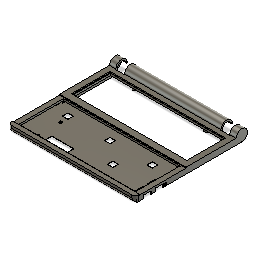
C_case (Autodesk Fusion 360 design; units mm, degrees)
Autodesk Fusion 360 part; units mm, degrees
sketch "Sketch1" plane through (0, 0, 0) normal (0, 1, 0) x (1, 0, 0)
  line L0 (0, 0) -> (230.6, 0)
  line L1 (230.6, 0) -> (230.6, 183)
  line L2 (230.6, 183) -> (0, 183)
  line L3 (0, 183) -> (0, 0)
  dimension "d1" = 230.6
  dimension "d2" = 183
  constraint horizontal L0
  constraint vertical L1
  constraint horizontal L2
  constraint vertical L3
  constraint coincident L0.start L3.end
  measures "d1" distance of L0.start L0.end
  measures "d2" distance of L0.start L2.end
extrude "Extrude1" add sketch "Sketch1" along normal blind 11
sketch "Sketch2" plane through (0, 11, 0) normal (0, 1, 0) x (-1, 0, 0)
  line L0 (0, 0) -> (-230.6, 0)
  line L1 (-230.6, -183) -> (0, -183)
  line L2 (-9, -10) -> (-221.6, -10)
  line L3 (-221.6, -10) -> (-221.6, -91.1)
  line L4 (-221.6, -91.1) -> (-9, -91.1)
  line L5 (-9, -91.1) -> (-9, -10)
  line L6 (-115.3, -77.3448) -> (-115.3, -22.2714) construction
  line L7 (0, -183) -> (0, 0)
  line L8 (-230.6, 0) -> (-230.6, -183)
  dimension "d5" = 212.6
  dimension "d6" = 81.1
  dimension "d7" = 10
  constraint horizontal L2
  constraint vertical L3
  constraint horizontal L4
  constraint vertical L5
  constraint perpendicular L1 L6
  constraint symmetric L3 L5 L6
  measures "d5" distance of L3.end L4.end
  measures "d6" distance of L2.start L4.end
  measures "d7" distance of L0 L2
extrude "Extrude2" cut sketch "Sketch2" against normal blind 5 contours L2 L3 L4 L5
sketch "Sketch3" plane through (0, 11, 0) normal (0, 1, 0) x (-1, 0, 0)
  line L0 (-221.6, -10) -> (-9, -10)
  line L1 (-9, -10) -> (-9, -91.1)
  line L2 (-9, -91.1) -> (-221.6, -91.1)
  line L3 (-221.6, -91.1) -> (-221.6, -10)
  line L4 (0, 0) -> (-230.6, 0)
  line L5 (-230.6, -183) -> (0, -183)
  line L6 (-10.05, -175) -> (-220.55, -175)
  line L7 (-220.55, -175) -> (-220.55, -104.5)
  line L8 (-220.55, -104.5) -> (-10.05, -104.5)
  line L9 (-10.05, -104.5) -> (-10.05, -175)
  line L10 (-115.3, -158.8) -> (-115.3, -113.8) construction
  line L11 (0, -183) -> (0, 0)
  line L12 (-230.6, 0) -> (-230.6, -183)
  dimension "d10" = 210.5
  dimension "d11" = 70.5
  dimension "d12" = 8
  constraint horizontal L6
  constraint vertical L7
  constraint horizontal L8
  constraint vertical L9
  constraint vertical L10
  constraint symmetric L7 L9 L10
  measures "d10" distance of L6.start L6.end
  measures "d11" distance of L6.start L8.end
  measures "d12" distance of L5 L6
extrude "Extrude3" cut sketch "Sketch3" against normal blind 1.95 contours L6 L7 L8 L9
sketch "Sketch4" plane through (0, 9.05, 0) normal (0, 1, 0) x (-1, 0, 0)
  line L0 (-10.05, -104.5) -> (-220.55, -104.5)
  line L1 (-220.55, -104.5) -> (-220.55, -175)
  line L2 (-220.55, -175) -> (-10.05, -175)
  line L3 (-10.05, -175) -> (-10.05, -104.5)
  line L4 (-11.55, -174.5) -> (-219.05, -174.5)
  line L5 (-219.05, -174.5) -> (-219.05, -105)
  line L6 (-219.05, -105) -> (-11.55, -105)
  line L7 (-11.55, -105) -> (-11.55, -174.5)
  dimension "d15" = 0.5
  dimension "d16" = 0.5
  dimension "d17" = 1.5
  dimension "d18" = 1.5
  constraint horizontal L4
  constraint vertical L5
  constraint horizontal L6
  constraint vertical L7
  measures "d15" distance of L2 L4
  measures "d16" distance of L0 L6
  measures "d17" distance of L3 L7
  measures "d18" distance of L1 L5
extrude "Extrude4" cut sketch "Sketch4" against normal blind 4.75 contours L4 L5 L6 L7
sketch "Sketch6" plane through (0, 0, 0) normal (-1, 0, 0) x (0, 0, 1)
  line L0 (-183, 0) -> (0, 0)
  line L1 (0, 0) -> (0, 11)
  line L2 (-183, 11) -> (-183, 0)
  line L3 (-8, 11) -> (-93, 11)
  line L4 (-93, 11) -> (-93, 9.5)
  line L5 (-93, 9.5) -> (-8, 9.5)
  line L6 (-8, 9.5) -> (-8, 11)
  line L7 (0, 11) -> (-183, 11)
  dimension "d26" = 1.5
  dimension "d27" = 85
  dimension "d28" = 8
  constraint horizontal L3
  constraint vertical L4
  constraint horizontal L5
  constraint vertical L6
  measures "d26" distance of L3.start L5.end
  measures "d27" distance of L3.start L3.end
  measures "d28" distance of L1 L6
extrude "Extrude6" cut sketch "Sketch6" against normal through all contours L3 L4 L5 L6 L7
sketch "Sketch8" plane through (0, 0, 0) normal (-1, 0, 0) x (0, 0, 1)
  line L0 (-183, 11) -> (-183, 0)
  line L1 (-183, 0) -> (0, 0)
  line L2 (0, 0) -> (0, 11)
  circle A0 centre (-194.5, 10.5) radius 10.5
  circle A1 centre (-194.5, 10.5) radius 9
  line L3 (-183, 0) -> (-194.5, 0)
  line L4 (-183, 0) -> (-184, 0)
  line L5 (-184, 0) -> (-184, 10.5)
  line L6 (-184, 10.5) -> (-183, 10.5)
  line L7 (-183, 10.5) -> (-183, 0)
  line L8 (-183, 11) -> (-184.0119, 11)
  line L9 (-93, 9.5) -> (-93, 11)
  line L10 (-93, 11) -> (-183, 11)
  line L11 (0, 11) -> (-8, 11)
  line L12 (-8, 11) -> (-8, 9.5)
  line L13 (-8, 9.5) -> (-93, 9.5)
  circle A2 centre (-194.5, 10.5) radius 7.5
  line L14 (-194.5, 10.5) -> (-203.5, 10.5)
  line L15 (-194.5, 10.5) -> (-202.7916, 14)
  dimension "d36" = 21
  dimension "d37" = 18
  dimension "d58" = 1
  dimension "d160" = 15
  dimension "d161" = 3.5
  constraint concentric A0 A1
  constraint coincident L0.end L1.start
  constraint coincident A0 L3.end
  constraint tangent A0 L3
  constraint parallel L1 L3
  constraint horizontal L4
  constraint vertical L5
  constraint horizontal L6
  constraint vertical L7
  constraint coincident A0 L5.end
  constraint tangent A0 L5
  constraint coincident L0.start L8.start
  constraint coincident A0 L8.end
  constraint perpendicular L0 L8
  constraint concentric A1 A2
  constraint coincident A0.centre A1.centre
  constraint coincident A1 L14.end
  constraint horizontal L14
  constraint coincident A1 L15.end
  measures "d36" diameter of A0
  measures "d37" diameter of A1
  measures "d58" distance of L5.end L6.end
  measures "d160" diameter of A2
  measures "d161" vertical distance of L14.end L15.end
extrude "Extrude7" add sketch "Sketch8" against normal blind 230.6 contours L0 A0 L6 L8 | L0 L3 L4 L5 L6 L7 | A0 | A1 A2 L14 L15 picked at (-186.0614, 9.6803)
extrude "Extrude8" add sketch "Sketch8" against normal blind 1.5 contours A0 L3 L5 | A1 A2 L14 L15 | A1 A2 L14 L15 | A2 L14 L15 | A2 L14 L15
sketch "Sketch9" plane through (230.6, 0, 0) normal (1, 0, 0) x (0, 0, -1)
  line L0 (183, 0) -> (194.5, 0)
  line L1 (0, 11) -> (0, 0)
  line L2 (0, 0) -> (184, 0)
  line L3 (184, 0) -> (184, 10.5)
  line L4 (184.0119, 11) -> (93, 11)
  circle A0 centre (194.5, 10.5) radius 10.5
  line L5 (184, 10.5) -> (184, 0)
  line L6 (184, 0) -> (194.5, 0)
  line L7 (184, 10.5) -> (184, 11)
  line L8 (184.0119, 11) -> (184, 11)
  line L9 (93, 11) -> (93, 9.5)
  line L10 (93, 9.5) -> (8, 9.5)
  line L11 (8, 9.5) -> (8, 11)
  line L12 (8, 11) -> (0, 11)
  arc A1 (184, 10.5) -> (184.0119, 11) centre (194.5, 10.5) ccw
  arc A2 (201.4096, 13.4167) -> (202, 10.5) centre (194.5, 10.5) ccw
  line L13 (201.4096, 13.4167) -> (202.7916, 14)
  line L14 (203.5, 10.5) -> (202, 10.5)
  point P0 (183, 11)
  constraint coincident L3.end A0
  constraint coincident L3.end L5.start
  constraint coincident L2.end L3.start
  constraint coincident L0.end L6.end
  constraint coincident L4 L7.end
  constraint tangent A0 L7
  constraint parallel L3 L7
  constraint coincident L4.start L8.start
extrude "Extrude9" add sketch "Sketch9" against normal blind 1.5 contours L0 L3 A0 L5 L6 A1 | A0 A1
sketch "Sketch5" plane through (0, 0, 0) normal (0, -1, 0) x (1, 0, 0)
  line L0 (0, 0) -> (0, -194.5)
  line L1 (230.6, -194.5) -> (230.6, 0)
  line L2 (230.6, 0) -> (0, 0)
  line L3 (1.5, -183) -> (229.1, -183)
  line L4 (229.1, -183) -> (229.1, -3.5)
  line L5 (229.1, -3.5) -> (1.5, -3.5)
  line L6 (1.5, -3.5) -> (1.5, -183)
  line L7 (1.5, -184) -> (229.1, -184)
  line L8 (229.1, -184) -> (229.1, -206)
  line L9 (229.1, -206) -> (1.5, -206)
  line L10 (1.5, -206) -> (1.5, -184)
  line L11 (229.1, -184) -> (229.1, -194.5)
  line L12 (219.1, -183) -> (203.1, -183)
  line L13 (203.1, -183) -> (203.1, -206)
  line L14 (203.1, -206) -> (219.1, -206)
  line L15 (219.1, -206) -> (219.1, -183)
  line L16 (11.5, -183) -> (27.5, -183)
  line L17 (27.5, -183) -> (27.5, -206)
  line L18 (27.5, -206) -> (11.5, -206)
  line L19 (11.5, -206) -> (11.5, -183)
  line L20 (1.5, -184) -> (229.1, -184)
  line L21 (0, -194.5) -> (1.5, -194.5)
  line L22 (1.5, -194.5) -> (1.5, -184)
  line L23 (229.1, -194.5) -> (230.6, -194.5)
  line L24 (1.5, -183) -> (1.5, -184)
  line L25 (229.1, -183) -> (229.1, -184)
  dimension "d21" = 1.5
  dimension "d22" = 1.5
  dimension "d23" = 3.5
  dimension "d44" = 22
  dimension "d51" = 10
  dimension "d52" = 16
  dimension "d53" = 10
  dimension "d54" = 16
  dimension "d59" = 1
  constraint horizontal L3
  constraint vertical L4
  constraint horizontal L5
  constraint vertical L6
  constraint horizontal L7
  constraint vertical L8
  constraint horizontal L9
  constraint vertical L10
  constraint coincident L7.start L10.end
  constraint collinear L4 L8
  constraint horizontal L12
  constraint vertical L13
  constraint horizontal L14
  constraint vertical L15
  constraint coincident L9 L13.end
  constraint coincident L3 L12.start
  constraint horizontal L16
  constraint vertical L17
  constraint horizontal L18
  constraint vertical L19
  constraint coincident L9 L17.end
  constraint coincident L3 L16.start
  constraint coincident L7.end L8.start
  measures "d21" distance of L0 L6
  measures "d22" distance of L1 L4
  measures "d23" distance of L2 L5
  measures "d44" distance of L7.end L8.end
  measures "d51" distance of L10 L19
  measures "d52" distance of L17.end L18.end
  measures "d53" distance of L8 L15
  measures "d54" distance of L13 L15
  measures "d59" distance of L3 L7
extrude "Extrude5" cut sketch "Sketch5" against normal blind 5.4 contours L3 L4 L5 L6 L12 L16
extrude "Extrude10" cut sketch "Sketch5" against normal blind 10.5 contours L7 L9 L10 L19 L20 L22 | L3 L7 L19 L20 L24 | L7 L8 L9 L11 L15 L20 | L7 L9 L17 L18 L19 L20 | L3 L7 L16 L17 L19 L20 | L3 L7 L15 L20 L25 | L7 L9 L13 L17 L20 | L3 L7 L13 L17 L20 | L7 L9 L13 L14 L15 L20 | L3 L7 L12 L13 L15 L20
sketch "Sketch11" plane through (0, 10.5, 0) normal (0, -1, 0) x (1, 0, 0)
  line L0 (229.1, -203.5) -> (1.5, -203.5)
  line L1 (229.1, -187) -> (229.1, -183)
  line L2 (229.1, -183) -> (1.5, -183)
  line L3 (1.5, -183) -> (1.5, -187)
  line L4 (1.5, -187) -> (229.1, -187)
  line L5 (229.1, -187) -> (229.1, -183)
  line L6 (229.1, -183) -> (1.5, -183)
  line L7 (1.5, -183) -> (1.5, -187)
  line L8 (1.5, -187) -> (229.1, -187)
  line L9 (1.5, -203.5) -> (1.5, -205)
  line L10 (1.5, -205) -> (229.1, -205)
  line L11 (229.1, -205) -> (229.1, -203.5)
  constraint horizontal L4
  constraint vertical L5
  constraint horizontal L6
  constraint vertical L7
  constraint coincident L1.end L2.start
  constraint coincident L3.end L4.start
extrude "Extrude13" add sketch "Sketch11" along normal up to surface (5.1 mm away) contours L1 L2 L3 L4 L5 L6 L7 L8
extrude "Extrude11" cut sketch "Sketch5" against normal through all contours L7 L9 L17 L18 L19 L20 | L3 L7 L16 L17 L19 L20 | L7 L9 L13 L14 L15 L20 | L3 L7 L12 L13 L15 L20
fillet "Fillet4" radius 6 tangency weight 1.013 2 edges at (230.6, 5.5, 0) (0, 5.5, 0)
sketch "Sketch22" plane through (0, 5.4, 0) normal (0, -1, 0) x (1, 0, 0)
  line L0 (219.1, -183) -> (219.1, -187)
  line L1 (219.1, -187) -> (229.1, -187)
  line L2 (229.1, -187) -> (229.1, -3.5)
  line L3 (229.1, -3.5) -> (1.5, -3.5)
  line L4 (1.5, -3.5) -> (1.5, -187)
  line L5 (1.5, -187) -> (11.5, -187)
  line L6 (11.5, -187) -> (11.5, -183)
  line L7 (11.5, -183) -> (27.5, -183)
  line L8 (27.5, -183) -> (27.5, -187)
  line L9 (27.5, -187) -> (203.1, -187)
  line L10 (203.1, -187) -> (203.1, -183)
  line L11 (203.1, -183) -> (219.1, -183)
  line L12 (219.05, -105) -> (219.05, -174.5)
  line L13 (219.05, -174.5) -> (11.55, -174.5)
  line L14 (11.55, -174.5) -> (11.55, -105)
  line L15 (11.55, -105) -> (219.05, -105)
  line L16 (11.5, -187) -> (10, -187)
  line L17 (10, -187) -> (10, -87)
  line L18 (10, -87) -> (11.5, -87)
  line L19 (11.5, -87) -> (11.5, -187)
  line L20 (219.1, -187) -> (220.6, -187)
  line L21 (220.6, -187) -> (220.6, -87)
  line L22 (220.6, -87) -> (219.1, -87)
  line L23 (219.1, -87) -> (219.1, -187)
  dimension "d170" = 1.5
  dimension "d171" = 100
  constraint horizontal L16
  constraint vertical L17
  constraint horizontal L18
  constraint vertical L19
  constraint coincident L5.end L6.start
  constraint horizontal L20
  constraint vertical L21
  constraint horizontal L22
  constraint vertical L23
  constraint coincident L0.end L1.start
  constraint equal L18 L22
  constraint equal L19 L23
  measures "d170" distance of L17.end L18.end
  measures "d171" distance of L16.end L17.end
extrude "Extrude24" add sketch "Sketch22" along normal blind 4 contours L0 L1 L20 L21 L22 L23 | L5 L6 L16 L17 L18 L19
sketch "Sketch12" plane through (0, 5.4, 0) normal (0, -1, 0) x (1, 0, 0)
  line L0 (219.1, -183) -> (219.1, -87)
  line L1 (220.6, -187) -> (229.1, -187)
  line L2 (229.1, -187) -> (229.1, -3.5)
  line L3 (229.1, -3.5) -> (1.5, -3.5)
  line L4 (1.5, -3.5) -> (1.5, -187)
  line L5 (11.5, -87) -> (11.5, -183)
  line L6 (11.5, -183) -> (27.5, -183)
  line L7 (27.5, -183) -> (27.5, -187)
  line L8 (27.5, -187) -> (203.1, -187)
  line L9 (203.1, -187) -> (203.1, -183)
  line L10 (203.1, -183) -> (219.1, -183)
  line L11 (219.05, -105) -> (219.05, -174.5)
  line L12 (219.05, -174.5) -> (11.55, -174.5)
  line L13 (11.55, -174.5) -> (11.55, -105)
  line L14 (11.55, -105) -> (219.05, -105)
  circle A0 centre (39.8, -13.5) radius 2.75
  circle A1 centre (39.8, -55.5) radius 2.75
  circle A2 centre (224.8, -33.5) radius 2.75
  line L15 (230.6, -6) -> (230.6, -194.5)
  line L16 (0, -194.5) -> (0, -6)
  circle A3 centre (39.8, -13.5) radius 1.75
  circle A4 centre (39.8, -55.5) radius 1.75
  circle A5 centre (224.8, -33.5) radius 1.75
  line L17 (1.5, -3.5) -> (229.1, -3.5)
  line L18 (220.6, -87) -> (220.6, -187)
  line L19 (1.5, -187) -> (10, -187)
  line L20 (10, -187) -> (10, -87)
  line L21 (10, -87) -> (11.5, -87)
  line L22 (219.1, -87) -> (220.6, -87)
  dimension "d64" = 5.8
  dimension "d65" = 39.8
  dimension "d66" = 39.8
  dimension "d67" = 5.5
  dimension "d68" = 5.5
  dimension "d69" = 5.5
  dimension "d70" = 3.5
  dimension "d71" = 3.5
  dimension "d72" = 3.5
  dimension "d73" = 10
  dimension "d74" = 42
  dimension "d110" = 22
  constraint concentric A0 A3
  constraint concentric A1 A4
  constraint concentric A2 A5
  measures "d64" distance of A2.centre L15
  measures "d65" distance of A0.centre L16
  measures "d66" distance of A1.centre L16
  measures "d67" diameter of A0
  measures "d68" diameter of A1
  measures "d69" diameter of A2
  measures "d70" diameter of A5
  measures "d71" diameter of A3
  measures "d72" diameter of A4
  measures "d73" distance of A0.centre L17
  measures "d74" distance of A1.centre A0.centre
  measures "d110" vertical distance of A2.centre A1.centre
extrude "Extrude14" add sketch "Sketch12" along normal blind 4 contours A0 | A1 | A2
sketch "Sketch13" plane through (0, 6, 0) normal (0, 1, 0) x (-1, 0, 0)
  line L0 (-9, -91.1) -> (-9, -10)
  line L1 (-9, -10) -> (-221.6, -10)
  line L2 (-221.6, -10) -> (-221.6, -91.1)
  line L3 (-221.6, -91.1) -> (-9, -91.1)
  line L4 (-54, -10) -> (-94, -10)
  line L5 (-94, -10) -> (-94, -25)
  line L6 (-94, -25) -> (-54, -25)
  line L7 (-54, -25) -> (-54, -10)
  line L8 (-32, -76.1) -> (-42, -76.1)
  line L9 (-42, -76.1) -> (-42, -66.1)
  line L10 (-42, -66.1) -> (-32, -66.1)
  line L11 (-32, -66.1) -> (-32, -76.1)
  line L12 (-109, -76.1) -> (-119, -76.1)
  line L13 (-119, -76.1) -> (-119, -66.1)
  line L14 (-119, -66.1) -> (-109, -66.1)
  line L15 (-109, -66.1) -> (-109, -76.1)
  line L16 (-186, -76.1) -> (-196, -76.1)
  line L17 (-196, -76.1) -> (-196, -66.1)
  line L18 (-196, -66.1) -> (-186, -66.1)
  line L19 (-186, -66.1) -> (-186, -76.1)
  line L20 (-149, -41.1) -> (-159, -41.1)
  line L21 (-159, -41.1) -> (-159, -31.1)
  line L22 (-159, -31.1) -> (-149, -31.1)
  line L23 (-149, -31.1) -> (-149, -41.1)
  dimension "d78" = 40
  dimension "d79" = 45
  dimension "d80" = 15
  dimension "d162" = 10
  dimension "d163" = 10
  dimension "d164" = 15
  dimension "d165" = 23
  dimension "d166" = 100
  dimension "d167" = 177
  dimension "d168" = 140
  dimension "d169" = 50
  constraint horizontal L4
  constraint vertical L5
  constraint horizontal L6
  constraint vertical L7
  constraint coincident L1 L4.start
  constraint horizontal L8
  constraint vertical L9
  constraint horizontal L10
  constraint vertical L11
  constraint horizontal L12
  constraint vertical L13
  constraint horizontal L14
  constraint vertical L15
  constraint horizontal L16
  constraint vertical L17
  constraint horizontal L18
  constraint vertical L19
  constraint horizontal L20
  constraint vertical L21
  constraint horizontal L22
  constraint vertical L23
  constraint equal L12 L15
  constraint equal L16 L19
  constraint equal L12 L16
  constraint equal L8 L12
  constraint equal L12 L20
  constraint equal L20 L23
  constraint collinear L8 L12
  constraint collinear L12 L16
  measures "d78" distance of L5.end L6.end
  measures "d79" distance of L0 L7
  measures "d80" distance of L4.start L6.end
  measures "d162" distance of L8.start L8.end
  measures "d163" distance of L8.start L10.end
  measures "d164" distance of L3 L8
  measures "d165" distance of L0 L11
  measures "d166" distance of L0 L15
  measures "d167" distance of L0 L19
  measures "d168" distance of L0 L23
  measures "d169" distance of L3 L20
extrude "Extrude15" cut sketch "Sketch13" against normal through all contours L1 L4 L5 L6 L7 | L8 L9 L10 L11 | L12 L13 L14 L15 | L16 L17 L18 L19 | L20 L21 L22 L23
sketch "Sketch14" plane through (0, 0, 0) normal (-1, 0, 0) x (0, 0, 1)
  line L0 (-6, 11) -> (-6, 0)
  line L1 (-6, 11) -> (-8, 11)
  line L2 (-8, 11) -> (-8, 9.5)
  line L3 (-8, 9.5) -> (-93, 9.5)
  line L4 (-93, 9.5) -> (-93, 11)
  line L5 (-93, 11) -> (-184.0119, 11)
  arc A0 (-184.0119, 11) -> (-194.5, 0) centre (-194.5, 10.5) ccw
  line L6 (-194.5, 0) -> (-6, 0)
  line L7 (-58, 3.8) -> (-46, 3.8)
  line L8 (-46, 3.8) -> (-46, 1.8)
  line L9 (-46, 1.8) -> (-58, 1.8)
  line L10 (-58, 1.8) -> (-58, 3.8)
  circle A1 centre (-36.6, 2.15) radius 2.75
  line L11 (-30.6, 4.3) -> (-22.5, 4.3)
  line L12 (-22.5, 4.3) -> (-22.5, 2.6)
  line L13 (-22.5, 2.6) -> (-24, 1.1)
  line L14 (-24, 1.1) -> (-29.1, 1.1)
  line L15 (-29.1, 1.1) -> (-30.6, 2.6)
  line L16 (-30.6, 2.6) -> (-30.6, 4.3)
  line L17 (-18.9, 4.75) -> (-12.8, 4.75)
  circle A2 centre (-18.9, 3) radius 1.75
  circle A3 centre (-12.8, 3) radius 1.75
  line L18 (-18.9, 1.25) -> (-12.8, 1.25)
  dimension "d82" = 12
  dimension "d83" = 2
  dimension "d84" = 1.8
  dimension "d85" = 40
  dimension "d86" = 5.5
  dimension "d87" = 30.6
  dimension "d88" = 2.15
  dimension "d89" = 6.8
  dimension "d90" = 16.5
  dimension "d91" = 8.1
  dimension "d92" = 3.2
  dimension "d93" = 5.2
  dimension "d94" = 1.7
  dimension "d95" = 135
  dimension "d96" = 135
  dimension "d99" = 3.5
  dimension "d100" = 1.25
  dimension "d101" = 6.1
  constraint horizontal L7
  constraint vertical L8
  constraint horizontal L9
  constraint vertical L10
  constraint parallel L3 L11
  constraint perpendicular L3 L12
  constraint parallel L3 L14
  constraint perpendicular L11 L16
  constraint horizontal L17
  constraint coincident L17.start A2
  constraint coincident L17.end A3
  constraint tangent L17 A3
  constraint coincident A2 L18.start
  constraint coincident A3 L18.end
  constraint tangent A3 L18
  constraint tangent A2 L18
  constraint tangent L17 A2
  constraint horizontal L18
  constraint equal L12 L16
  measures "d82" distance of L7.start L7.end
  measures "d83" distance of L7.start L9.end
  measures "d84" distance of L6 L9
  measures "d85" distance of L0 L8
  measures "d86" diameter of A1
  measures "d87" distance of L0 A1.centre
  measures "d88" distance of L6 A1.centre
  measures "d89" distance of L0 A3.centre
  measures "d90" distance of L0 L12
  measures "d91" distance of L11.start L11.end
  measures "d92" distance of L11 L14
  measures "d93" distance of L3 L11
  measures "d94" distance of L11.end L12.end
  measures "d95" angle of L15 L16
  measures "d96" angle of L12 L13
  measures "d99" diameter of A3
  measures "d100" distance of L6 L18
  measures "d101" distance of A2.centre A3.centre
extrude "Extrude16" cut sketch "Sketch14" against normal blind 14 contours L6 A1 | L7 L8 L9 L10 | L11 L12 L13 L14 L15 L16 | L17 A2 A3 L18 | A2 | A3 picked at (-36.5315, 1.6308)
sketch "Sketch15" plane through (230.6, 0, 0) normal (1, 0, 0) x (0, 0, -1)
  line L0 (6, 0) -> (6, 11)
  line L1 (6, 0) -> (194.5, 0)
  arc A0 (194.5, 0) -> (184.0119, 11) centre (194.5, 10.5) ccw
  line L2 (184.0119, 11) -> (93, 11)
  line L3 (93, 11) -> (93, 9.5)
  line L4 (93, 9.5) -> (8, 9.5)
  line L5 (8, 9.5) -> (8, 11)
  line L6 (15.8, 5.6) -> (29.3, 5.6)
  line L7 (29.3, 5.6) -> (29.3, 0)
  line L8 (29.3, 0) -> (15.8, 0)
  line L9 (15.8, 0) -> (15.8, 5.6)
  line L10 (37.8, 0) -> (51.3, 0)
  line L11 (51.3, 0) -> (51.3, 5.6)
  line L12 (51.3, 5.6) -> (37.8, 5.6)
  line L13 (37.8, 5.6) -> (37.8, 0)
  line L14 (54, 4.5) -> (57.5, 4.5)
  line L15 (57.5, 4.5) -> (57.5, 1)
  line L16 (57.5, 1) -> (54, 1)
  line L17 (54, 1) -> (54, 4.5)
  line L18 (8, 11) -> (6, 11)
  dimension "d102" = 13.5
  dimension "d103" = 13.5
  dimension "d104" = 5.6
  dimension "d105" = 5.6
  dimension "d106" = 22
  dimension "d107" = 9.8
  dimension "d122" = 3.5
  dimension "d123" = 3.5
  dimension "d124" = 2.7
  dimension "d125" = 1
  constraint horizontal L6
  constraint vertical L7
  constraint horizontal L8
  constraint vertical L9
  constraint coincident L1 L7.end
  constraint horizontal L10
  constraint vertical L11
  constraint horizontal L12
  constraint vertical L13
  constraint coincident L1 L10.start
  constraint horizontal L14
  constraint vertical L15
  constraint horizontal L16
  constraint vertical L17
  measures "d102" distance of L6.start L6.end
  measures "d103" distance of L11.end L12.end
  measures "d104" distance of L10.start L12.end
  measures "d105" distance of L6.start L8.end
  measures "d106" distance of L7 L11
  measures "d107" distance of L0 L9
  measures "d122" distance of L14.start L14.end
  measures "d123" distance of L14.start L16.end
  measures "d124" distance of L11 L17
  measures "d125" distance of L1 L16
extrude "Extrude17" cut sketch "Sketch15" against normal blind 14.5 contours L1 L6 L7 L8 L9 | L1 L10 L11 L12 L13 | L14 L15 L16 L17
sketch "Sketch16" plane through (0, 0, -10) normal (0, 0, -1) x (-1, 0, 0)
  line L0 (-9, 9.5) -> (-221.6, 9.5)
  line L1 (-221.6, 9.5) -> (-221.6, 6)
  line L2 (-221.6, 6) -> (-94, 6)
  line L3 (-94, 6) -> (-94, 5.4)
  line L4 (-94, 5.4) -> (-54, 5.4)
  line L5 (-54, 5.4) -> (-54, 6)
  line L6 (-54, 6) -> (-9, 6)
  line L7 (-9, 6) -> (-9, 9.5)
  line L8 (-28.6, 6) -> (-39.6, 6)
  line L9 (-39.6, 6) -> (-39.6, 8.5)
  line L10 (-39.6, 8.5) -> (-28.6, 8.5)
  line L11 (-28.6, 8.5) -> (-28.6, 6)
  line L12 (-120.1, 6) -> (-131.1, 6)
  line L13 (-131.1, 6) -> (-131.1, 8.5)
  line L14 (-131.1, 8.5) -> (-120.1, 8.5)
  line L15 (-120.1, 8.5) -> (-120.1, 6)
  line L16 (-191.1, 6) -> (-202.1, 6)
  line L17 (-202.1, 6) -> (-202.1, 8.5)
  line L18 (-202.1, 8.5) -> (-191.1, 8.5)
  line L19 (-191.1, 8.5) -> (-191.1, 6)
  dimension "d111" = 11
  dimension "d112" = 11
  dimension "d113" = 11
  dimension "d114" = 19.5
  dimension "d115" = 60
  dimension "d116" = 80.5
  dimension "d117" = 2.5
  dimension "d118" = 2.5
  dimension "d119" = 2.5
  constraint horizontal L8
  constraint vertical L9
  constraint horizontal L10
  constraint vertical L11
  constraint coincident L6 L8.start
  constraint horizontal L12
  constraint vertical L13
  constraint horizontal L14
  constraint vertical L15
  constraint coincident L2 L12.start
  constraint horizontal L16
  constraint vertical L17
  constraint horizontal L18
  constraint vertical L19
  constraint coincident L2 L16.start
  measures "d111" distance of L17.end L18.end
  measures "d112" distance of L13.end L14.end
  measures "d113" distance of L9.end L10.end
  measures "d114" distance of L1 L16.end
  measures "d115" distance of L13 L19
  measures "d116" distance of L9 L15
  measures "d117" distance of L16.end L17.end
  measures "d118" distance of L12.end L13.end
  measures "d119" distance of L8.end L9.end
extrude "Extrude18" cut sketch "Sketch16" against normal blind 2 contours L6 L8 L9 L10 L11 | L2 L16 L17 L18 L19 | L2 L12 L13 L14 L15
sketch "Sketch17" plane through (0, 0, 0) normal (0, -1, 0) x (1, 0, 0)
  line L0 (230.6, -51.3) -> (229.1, -51.3)
  line L1 (229.1, -51.3) -> (229.1, -194.5)
  line L2 (229.1, -194.5) -> (230.6, -194.5)
  line L3 (230.6, -194.5) -> (230.6, -51.3)
  line L4 (229.1, -53) -> (229.9, -53)
  line L5 (229.9, -53) -> (229.9, -58.5)
  line L6 (229.9, -58.5) -> (229.1, -58.5)
  line L7 (229.1, -58.5) -> (229.1, -53)
  dimension "d126" = 5.5
  dimension "d127" = 0.8
  dimension "d128" = 1.7
  constraint horizontal L4
  constraint vertical L5
  constraint horizontal L6
  constraint vertical L7
  constraint coincident L1 L4.start
  measures "d126" distance of L4.end L5.end
  measures "d127" distance of L4.start L4.end
  measures "d128" distance of L0 L4
extrude "Extrude19" cut sketch "Sketch17" against normal blind 5 contours L1 L4 L5 L6 L7
sketch "Sketch18" plane through (0, 5.4, 0) normal (0, -1, 0) x (1, 0, 0)
  circle A0 centre (224.8, -33.5) radius 2.75
  circle A1 centre (39.8, -13.5) radius 2.75
  line L0 (229.1, -29.3) -> (216.1, -29.3)
  line L1 (216.1, -29.3) -> (216.1, -15.8)
  line L2 (216.1, -15.8) -> (229.1, -15.8)
  line L3 (229.1, -15.8) -> (229.1, -3.5)
  line L4 (229.1, -3.5) -> (1.5, -3.5)
  line L5 (1.5, -3.5) -> (1.5, -187)
  line L6 (1.5, -187) -> (10, -187)
  line L7 (11.5, -87) -> (11.5, -183)
  line L8 (11.5, -183) -> (27.5, -183)
  line L9 (27.5, -183) -> (27.5, -187)
  line L10 (27.5, -187) -> (203.1, -187)
  line L11 (203.1, -187) -> (203.1, -183)
  line L12 (203.1, -183) -> (219.1, -183)
  line L13 (219.1, -183) -> (219.1, -87)
  line L14 (220.6, -187) -> (229.1, -187)
  line L15 (229.1, -187) -> (229.1, -51.3)
  line L16 (229.1, -51.3) -> (216.1, -51.3)
  line L17 (216.1, -51.3) -> (216.1, -37.8)
  line L18 (216.1, -37.8) -> (229.1, -37.8)
  line L19 (229.1, -37.8) -> (229.1, -29.3)
  line L20 (219.05, -105) -> (219.05, -174.5)
  line L21 (219.05, -174.5) -> (11.55, -174.5)
  line L22 (11.55, -174.5) -> (11.55, -105)
  line L23 (11.55, -105) -> (219.05, -105)
  circle A2 centre (39.8, -55.5) radius 2.75
  line L24 (94, -25) -> (54, -25)
  line L25 (54, -25) -> (54, -10)
  line L26 (54, -10) -> (94, -10)
  line L27 (94, -10) -> (94, -25)
  circle A3 centre (6, -7) radius 1.75
  circle A4 centre (6, -80) radius 1.75
  circle A5 centre (6, -150) radius 1.75
  line L28 (6, 0) -> (224.6, 0)
  line L29 (0, -194.5) -> (0, -38.3146)
  circle A6 centre (6, -7) radius 3.5
  circle A7 centre (6, -80) radius 3.5
  circle A8 centre (6, -150) radius 3.5
  line L30 (115.3, 16.8272) -> (115.3, -220) construction
  line L31 (230.6, -51.3) -> (230.6, -194.5)
  circle A9 centre (224.6, -7) radius 1.75
  circle A10 centre (224.6, -7) radius 3.5
  circle A11 centre (224.6, -80) radius 1.75
  circle A12 centre (224.6, -80) radius 3.5
  circle A13 centre (224.6, -150) radius 1.75
  circle A14 centre (224.6, -150) radius 3.5
  circle A15 centre (50, -180) radius 3.5
  circle A16 centre (50, -180) radius 1.75
  circle A17 centre (180.6, -180) radius 1.75
  circle A18 centre (180.6, -180) radius 3.5
  line L32 (1.5, -9.5) -> (229.1, -9.5)
  line L33 (149, -41.1) -> (149, -31.1)
  line L34 (149, -31.1) -> (159, -31.1)
  line L35 (159, -31.1) -> (159, -41.1)
  line L36 (159, -41.1) -> (149, -41.1)
  line L37 (186, -76.1) -> (186, -66.1)
  line L38 (186, -66.1) -> (196, -66.1)
  line L39 (196, -66.1) -> (196, -76.1)
  line L40 (196, -76.1) -> (186, -76.1)
  line L41 (32, -76.1) -> (32, -66.1)
  line L42 (32, -66.1) -> (42, -66.1)
  line L43 (42, -66.1) -> (42, -76.1)
  line L44 (42, -76.1) -> (32, -76.1)
  line L45 (109, -76.1) -> (109, -66.1)
  line L46 (109, -66.1) -> (119, -66.1)
  line L47 (119, -66.1) -> (119, -76.1)
  line L48 (119, -76.1) -> (109, -76.1)
  line L49 (10, -187) -> (10, -87)
  line L50 (10, -87) -> (11.5, -87)
  line L51 (219.1, -87) -> (220.6, -87)
  line L52 (220.6, -87) -> (220.6, -187)
  dimension "d131" = 7
  dimension "d132" = 80
  dimension "d133" = 150
  dimension "d134" = 6
  dimension "d135" = 6
  dimension "d136" = 6
  dimension "d137" = 3.5
  dimension "d138" = 7
  dimension "d157" = 180
  dimension "d158" = 44
  dimension "d159" = 6
  constraint equal A3 A4
  constraint equal A4 A5
  constraint concentric A3 A6
  constraint concentric A4 A7
  constraint concentric A5 A8
  constraint equal A6 A7
  constraint equal A7 A8
  constraint perpendicular L23 L30
  constraint symmetric A3 L30 A9
  constraint symmetric A4 L30 A11
  constraint symmetric A5 L30 A13
  constraint symmetric A6 L30 A10
  constraint symmetric A7 L30 A12
  constraint symmetric A8 L30 A14
  constraint concentric A15 A16
  constraint equal A8 A15
  constraint equal A5 A16
  constraint symmetric L30 A15 A18
  constraint symmetric L30 A16 A17
  constraint coincident L5 L32.start
  constraint coincident L3 L32.end
  constraint perpendicular L3 L32
  measures "d131" distance of A3.centre L28
  measures "d132" distance of A4.centre L28
  measures "d133" distance of A5.centre L28
  measures "d134" distance of A3.centre L29
  measures "d135" distance of A4.centre L29
  measures "d136" distance of A5.centre L29
  measures "d137" diameter of A3
  measures "d138" diameter of A6
  measures "d157" distance of L28 A15.centre
  measures "d158" horizontal distance of A5.centre A15.centre
  measures "d159" distance of L4 L32
extrude "Extrude20" add sketch "Sketch18" along normal up to surface (5.4 mm away) contours A10 L32 | A6 L32 | A7 | A8 | A12 | A14 | A15 | A18 picked at (224.5564, -9.2484) picked at (5.9564, -9.2484)
sketch "Sketch19" plane through (0, 0, 0) normal (-1, 0, 0) x (0, 0, 1)
  arc A0 (-34.8854, 0) -> (-38.3146, 0) centre (-36.6, 2.15) ccw
  line L0 (-34.8854, 0) -> (-6, 0)
  line L1 (-6, 11) -> (-6, 0)
  line L2 (-6, 11) -> (-8, 11)
  line L3 (-8, 11) -> (-8, 9.5)
  line L4 (-8, 9.5) -> (-93, 9.5)
  line L5 (-93, 9.5) -> (-93, 11)
  line L6 (-93, 11) -> (-184.0119, 11)
  arc A1 (-184.0119, 11) -> (-194.5, 0) centre (-194.5, 10.5) ccw
  line L7 (-194.5, 0) -> (-38.3146, 0)
  line L8 (-12.8, 1.25) -> (-18.9, 1.25)
  arc A2 (-18.9, 4.75) -> (-18.9, 1.25) centre (-18.9, 3) ccw
  line L9 (-18.9, 4.75) -> (-12.8, 4.75)
  arc A3 (-12.8, 1.25) -> (-12.8, 4.75) centre (-12.8, 3) ccw
  line L10 (-46, 3.8) -> (-46, 1.8)
  line L11 (-46, 1.8) -> (-58, 1.8)
  line L12 (-58, 1.8) -> (-58, 3.8)
  line L13 (-58, 3.8) -> (-46, 3.8)
  line L14 (-24, 1.1) -> (-29.1, 1.1)
  line L15 (-29.1, 1.1) -> (-30.6, 2.6)
  line L16 (-30.6, 2.6) -> (-30.6, 4.3)
  line L17 (-30.6, 4.3) -> (-22.5, 4.3)
  line L18 (-22.5, 4.3) -> (-22.5, 2.6)
  line L19 (-22.5, 2.6) -> (-24, 1.1)
  circle A4 centre (-7.75, 6.25) radius 7.75
  line L20 (0, -1.5) -> (-9.8878, -1.5)
  line L21 (0, 6.25) -> (0, -1.5)
  line L22 (0, 0) -> (0, 11)
  dimension "d141" = 15.5
  dimension "d143" = 1.5
  constraint horizontal L20
  constraint tangent A4 L20
  constraint coincident A4 L21.start
  constraint vertical L21
  constraint tangent A4 L21
  constraint collinear L21 L22
  measures "d141" diameter of A4
  measures "d143" distance of L0 L20
extrude "Extrude21" cut sketch "Sketch19" against normal through all contours A4 L20 L21 L22
sketch "Sketch20" plane through (0, 0, 0) normal (0, -1, 0) x (1, 0, 0)
  line L0 (1.5, -38.3146) -> (0, -38.3146)
  line L1 (0, -38.3146) -> (0, -194.5)
  line L2 (0, -194.5) -> (1.5, -194.5)
  line L3 (1.5, -194.5) -> (1.5, -38.3146)
  circle A0 centre (-3.5, -52) radius 4.5
  line L4 (224.6, 0) -> (6, 0)
  dimension "d144" = 52
  dimension "d145" = 9
  dimension "d146" = 3.5
  measures "d144" distance of A0.centre L4
  measures "d145" diameter of A0
  measures "d146" distance of L1 A0.centre
extrude "Extrude22" cut sketch "Sketch20" against normal blind 5.5 contours L1 A0 picked at (0.117, -52.776)
